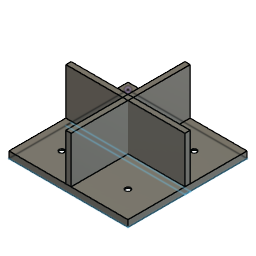
Kreuz (Autodesk Fusion 360 design; units mm, degrees)
Autodesk Fusion 360 part; units mm, degrees
sketch "Skizze1" plane through (0, 0, 0) normal (0, 1, 0) x (1, 0, 0)
  line L0 (0, 0) -> (90, 0)
  line L1 (90, 0) -> (90, -90)
  line L2 (90, -90) -> (0, -90)
  line L3 (0, -90) -> (0, 0)
  line L4 (0, -43) -> (90, -43)
  line L5 (90, -43) -> (90, -47)
  line L6 (90, -47) -> (0, -47)
  line L7 (0, -47) -> (0, -43)
  constraint horizontal L0
  constraint vertical L1
  constraint horizontal L2
  constraint vertical L3
  constraint coincident L0.start L3.end
  constraint horizontal L4
  constraint vertical L5
  constraint horizontal L6
  constraint vertical L7
  constraint coincident L1 L5.end
  constraint coincident L3 L4.start
extrude "Extrusion1" add sketch "Skizze1" along normal blind 5 makes body 1
extrude "Extrusion2" add sketch "Skizze1" along normal blind 35 separate body contours L1 L3 L4 L5 L6 L7 makes body 2
move_body "Verschieben2" bodies 2 to x (1, 0, 0) y (0, 1, 0) z (0, 0, 1) at (0, 5, 0)
sketch "Skizze2" plane through (0, 0, 0) normal (0, 1, 0) x (1, 0, 0)
copy_body "Körper kopieren/einfügen2" bodies 2 makes body 3
move_body "Verschieben5" bodies 3 to x (1, 0, 0) y (0, 1, 0) z (0, 0, 1) at (0, 0, 0)
move_body "Verschieben6" bodies 3 to x (0, 0, 1) y (0, 1, 0) z (-1, 0, 0) at (90, 0, 0)
sketch "Skizze3" plane through (0, 0, 0) normal (0, 1, 0) x (1, 0, 0)
sketch "Skizze4" plane through (0, 5, 0) normal (0, 1, 0) x (-1, 0, 0)
  line L0 (0, 90) -> (-90, 90)
  line L1 (-90, 90) -> (-90, 0)
  line L2 (-90, 0) -> (0, 0)
  line L3 (0, 0) -> (0, 90)
  circle A0 centre (-20, 20) radius 2
  circle A1 centre (-70, 20) radius 2
  circle A2 centre (-20, 70) radius 2
  circle A3 centre (-70, 70) radius 2
hole "Bohrung1" at (20, 5, 70) at (20, 5, 20) at (70, 5, 20) at (70, 5, 70) direction (0, -1, 0) diameter 4 end through all bodies 1
sketch "Skizze5" plane through (0, 0, 0) normal (0, 1, 0) x (1, 0, 0)
  line L0 (13, -80) -> (43, -80)
  line L1 (43, -80) -> (43, -60)
  line L2 (43, -60) -> (13, -60)
  line L3 (13, -60) -> (13, -80)
  line L4 (13, -80) -> (80, -80)
  line L5 (80, -80) -> (80, -10)
  line L6 (80, -10) -> (13, -10)
  line L7 (13, -10) -> (13, -80)
  constraint horizontal L0
  constraint vertical L1
  constraint horizontal L2
  constraint vertical L3
  constraint horizontal L4
  constraint vertical L5
  constraint horizontal L6
  constraint vertical L7
extrude "Extrusion3" cut sketch "Skizze5" along normal blind 4 contours L1 L2 L4 L5 L6 L7 bodies 1
sketch "Skizze6" plane through (0, 0, 0) normal (0, 1, 0) x (1, 0, 0)
  line L0 (43, -80) -> (13, -80)
  line L1 (13, -80) -> (13, -60)
  line L2 (13, -60) -> (43, -60)
  line L3 (43, -60) -> (43, -80)
  constraint horizontal L0
  constraint vertical L1
  constraint horizontal L2
  constraint vertical L3
extrude "Extrusion4" cut sketch "Skizze6" along normal blind 4 bodies 1
move_body "Verschieben3" [rolled back]
move_body "Verschieben4" [rolled back]
move_body "Verschieben1" [rolled back]
pasted_body "Körper kopieren/einfügen1" makes body 4
